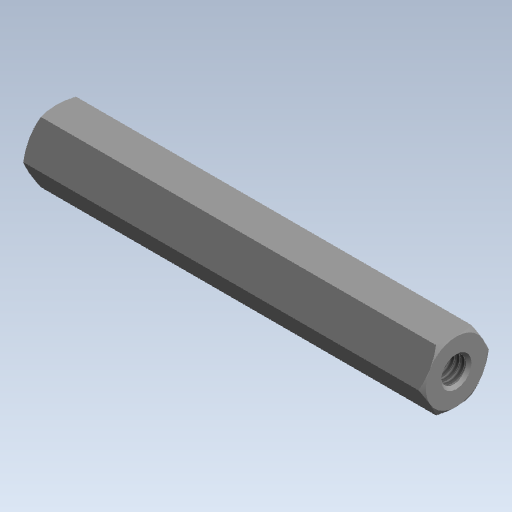
# Autodesk Inventor part: SLSBF6-39.5-M3-N3
Saved by Autodesk Inventor 2020 (Build 240168000, 168)
## iProperties
Part Number: SLSBF6-39.5-M3-N3
Material: 一般
Catalog Web Link: https://jp.misumi-ec.com/vona2/detail/110300206620/?HissuCode=SLSBF6-39.5-M3-N3
Description: 既製品
Vendor: MISUMI
Document SubType Name: Modeling
Designer: partserver
Manufacturer: MISUMI
Mass: 8.6 g
Surface Area: 10.0772 cm^2
Volume: 1.14942 cm^3
Density: 7.48201 g/cm^3
Appearance: PSOLRGB-175-175-175
Category: PARTsolutions
Company: MISUMI
PSOL_IDENT_0: {$CADENAS_DATA\23d-libs\misumi\metric\19_posts_stands\plsbf.prj},253 {VTYP=3D},{NB=SLSBF6-39.5-M3-N3
PSOL_IDENT_1: },{LINA=SLSBF6-39.5-M3-N3},{NN=NLSBF, LSBF, PLSBF, BLSBF, SLSBF, ALSBF, ABLSBF},{DATE=20.04.2021 01:
PSOL_IDENT_2: 53:51},{GEOMDATE=25.03.2021 00:56:23},{VERSION=},{LINEID=230},{WBVAR=MAT,ST,M,N,ALT1,L,ALT4,ALT2,ALT
PSOL_IDENT_3: 3},{WBNUMERIC=M,N,L}  {NB=SLSBF6-39.5-M3-N3},{LINA=SLSBF6-39.5-M3-N3},{KT=DUMMY},{PN=SLSBF6-39.5-M3-
PSOL_IDENT_4: N3},{TYPE=SLSBF},{MAT=304},{MATALG= 'LCS','Low Carbon Steel','304','SUS304','A2011','A2011 Aluminum
PSOL_IDENT_5: Alloy' },{ST=-},{STALG= '-','-' },{B=6},{M=3},{MALG=[3,4]},{N=3},{NALG=[3,4]},{ALT1=},{L=39.5},{LALG=
PSOL_IDENT_6: [15:100/0.5]},{LMIN=15},{LMIN1=12},{LMIN1ALG=12},{LMIN2=15.000},{C=6.9},{ALT4=},{ALT4ALG= '', 'w/o L
PSOL_IDENT_7: VC (L Dimension Accuracy Change)', 'LVC', 'with LVC (L Dimension Accuracy Change)'},{ALT4PN=},{ALT2=
PSOL_IDENT_8: },{ALT2ALG='','w/o MD (Left End Change The Effective Tap Depth)','MD','with MD (Left End Change The
PSOL_IDENT_9: Effective Tap Depth)'},{ALT2PN=},{ALT3=},{ALT3ALG='','w/o ND (Right End Change The Effective Tap Dep
PSOL_IDENT_10: th)','ND','with ND (Right End Change The Effective Tap Depth)'},{ALT3PN=},{MAV=3},{MPITCH=0.5},{NPIT
PSOL_IDENT_11: CH=0.5},{NDEPT=9},{MDEPT=9},{M3D=6},{N3D=6}
NB: SLSBF6-39.5-M3-N3
NN: NLSBF, LSBF, PLSBF, BLSBF, SLSBF, ALSBF, ABLSBF
NT: Hex Posts - Both Ends Tapped - L Dimension, Thread Dia. Configurable -
NBSYN: $PN.
LINA: SLSBF6-39.5-M3-N3
CATALOG: Misumi
PN: SLSBF6-39.5-M3-N3
MAT: SUS304
ST: -
B: 6
M: 3
N: 3
ALT1: w/o LKC (L Dimension Tolerance)
L: 39.5
C: 6.9
ALT4: w/o LVC (L Dimension Accuracy Change)
ALT2: w/o MD (Left End Change The Effective Tap Depth)
ALT3: w/o ND (Right End Change The Effective Tap Depth)
SUPPLIER: MISUMI
ARTICLENO: SLSBF6-39.5-M3-N3
BOMINFO: SLSBF6-39.5-M3-N3
CREATOR: CADENAS GmbH
Title: SLSBF6-39.5-M3-N3
Author: Cadenas PARTsolutions
Autodesk Inventor part; units mm, degrees
sketch "Sketch_1" plane through (0, 0, 0) normal (0, 0, 1) x (1, 0, 0)
  line L0 (39.5, 0) -> (0, 0)
  line L1 (0, 0) -> (0, 3)
  line L2 (0, 3) -> (0.5485, 3.95)
  line L3 (0.5485, 3.95) -> (38.9515, 3.95)
  line L4 (38.9515, 3.95) -> (39.5, 3)
  line L5 (39.5, 3) -> (39.5, 0)
  line L6 (39.5, 0) -> (0, 0)
  constraints: 14 end point
revolve "Revolution1" add sketch "Sketch_1" angle 360 about axis through (39.5, 0, 0) along (1, 0, 0)
sketch "Sketch_2" plane through (0, 0, 0) normal (1, 0, 0) x (0, 1, 0)
  line L0 (6, 6) -> (-6, 6)
  line L1 (-6, 6) -> (-6, -6)
  line L2 (-6, -6) -> (6, -6)
  line L3 (6, -6) -> (6, 6)
  line L4 (-1.7321, 3) -> (-3.4641, 0)
  line L5 (-3.4641, 0) -> (-1.7321, -3)
  line L6 (-1.7321, -3) -> (1.7321, -3)
  line L7 (1.7321, -3) -> (3.4641, 0)
  line L8 (3.4641, 0) -> (1.7321, 3)
  line L9 (1.7321, 3) -> (-1.7321, 3)
  constraints: 20 end point
extrude "Extrusion1" cut sketch "Sketch_2" along normal blind 39.5
sketch "Sketch3" plane through (0, 0, 0) normal (-1, 0, 0) x (0, 0, 1)
  point P0 (0, 0)
hole "Hole1" at (0, 0, 0) direction (1, 0, 0) diameter 2.459 depth 8.2901 tip angle 120 countersink diameter 3 countersink angle 90 thread size "M3x0.5" class "6H" standard "ISO Metric profile"
sketch "Sketch4" plane through (39.5, 0, 0) normal (1, 0, 0) x (0, 0, -1)
  point P0 (0, 0)
hole "Hole2" at (39.5, 0, 0) direction (-1, 0, 0) diameter 2.459 depth 8.2901 tip angle 120 countersink diameter 3 countersink angle 90 thread size "M3x0.5" class "6H" standard "ISO Metric profile"
ref_plane "C3_XY" through (39.5, 0, 0) normal (-1, 0, 0) x (0, 0, -1)
ref_plane "C3_YZ" through (39.5, 0, 0) normal (0, 0, -1) x (0, -1, 0)
ref_plane "C3_ZX" through (39.5, 0, 0) normal (0, -1, 0) x (-1, 0, 0)
body "Solid1"
